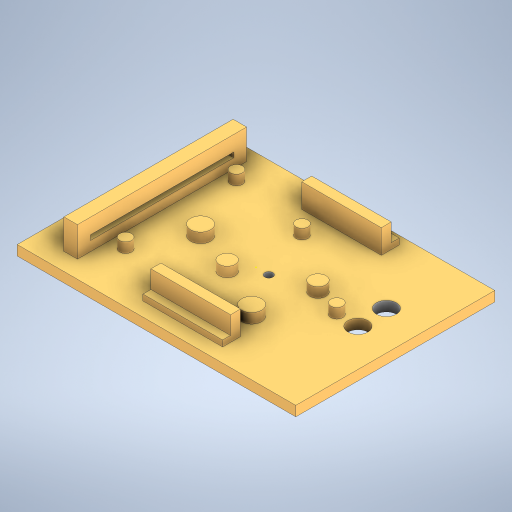
# Autodesk Inventor part: Base
Saved by Autodesk Inventor 2024 (Build 280153000, 153)
## iProperties
Created: 2024-04-22
Part Number: Base
Material: Generic
Document SubType Name: Modeling
Designer: samue
Density: 1 g/cm^3
Appearance: Default
Author: samue
Autodesk Inventor part; units mm, degrees
ref_plane "YZ Plane" through (0, 0, 0) normal (1, 0, 0) x (0, 1, 0)
ref_plane "XZ Plane" through (0, 0, 0) normal (0, 1, 0) x (-1, 0, 0)
ref_plane "XY Plane" through (0, 0, 0) normal (0, 0, 1) x (1, 0, 0)
sketch "Sketch1" plane through (0, 0, 0) normal (0, 1, 0) x (-1, 0, 0)
  line L0 (70, 50) -> (-70, 50)
  line L1 (-70, 50) -> (-70, -50)
  line L2 (-70, -50) -> (70, -50)
  line L3 (70, -50) -> (70, 50)
  line L4 (70, 50) -> (-70, -50) construction
  line L5 (-70, 50) -> (70, -50) construction
  point P0 (0, 0)
  dimension "d0" = 140
  dimension "d1" = 100
  constraints: 12 end point, 2 midpoint, 2 parallel, 1 horizontal, 1 perpendicular
  measures "d0" distance of L2.end L1.end
  measures "d1" distance of L0.end L1.end
extrude "Extrusion1" add sketch "Sketch1" along normal blind 5
sketch "Sketch2" plane through (0, 5, 0) normal (0, 1, 0) x (1, 0, 0)
  circle A0 centre (-42.6045, 32.7902) radius 3
  circle A1 centre (-41.0016, -24.5315) radius 3
  circle A2 centre (-27.8394, 0) radius 5
  circle A3 centre (-2.5867, 25.6769) radius 3
  circle A4 centre (-5.5867, -8.8777) radius 4
  circle A5 centre (19.9874, -22.1936) radius 5
  circle A6 centre (26.1305, 5) radius 4
  circle A7 centre (40.6174, 0) radius 3
  point P0 (0, 0)
  dimension "d4" = 6
  dimension "d5" = 6
  dimension "d6" = 10
  dimension "d7" = 6
  dimension "d8" = 8
  dimension "d9" = 10
  dimension "d12" = 8
  dimension "d13" = 6
  constraints: 8 centre point
  measures "d4" diameter of A0
  measures "d5" diameter of A1
  measures "d6" diameter of A2
  measures "d7" diameter of A3
  measures "d8" diameter of A4
  measures "d9" diameter of A5
  measures "d12" diameter of A6
  measures "d13" diameter of A7
extrude "Extrusion2" add sketch "Sketch2" along normal blind 5
sketch "Sketch3" plane through (0, 5, 0) normal (0, 1, 0) x (1, 0, 0)
  line L0 (-55.5, 43.7813) -> (-48.5, 43.7813)
  line L1 (-48.5, 43.7813) -> (-48.5, -41.2187)
  line L2 (-48.5, -41.2187) -> (-55.5, -41.2187)
  line L3 (-55.5, -41.2187) -> (-55.5, 43.7813)
  line L4 (-70, 50) -> (-70, -50) projected
  point P0 (0, 0)
  dimension "d14" = 7
  dimension "d15" = 85
  dimension "d18" = 21.5
  constraints: 8 end point, 2 parallel, 1 horizontal, 1 perpendicular
  measures "d14" distance of L1.end L2.end
  measures "d15" distance of L0.end L1.end
  measures "d18" distance between parallel lines of L4 L1
extrude "Extrusion3" add sketch "Sketch3" along normal blind 15
sketch "Sketch4" plane through (-48.5, 5, 41.2187) normal (1, 0, 0) x (0, 0, -1)
  line L0 (6.5, 4.85) -> (78.5, 4.85)
  line L1 (78.5, 4.85) -> (78.5, 7.35)
  line L2 (78.5, 7.35) -> (6.5, 7.35)
  line L3 (6.5, 7.35) -> (6.5, 4.85)
  line L4 (85, 0) -> (0, 0) projected
  line L5 (0, 0) -> (0, 15) projected
  point P0 (41.2187, -5)
  dimension "d19" = 2.5
  dimension "d20" = 4.85
  dimension "d23" = 72
  dimension "d24" = 6.5
  constraints: 8 end point, 2 parallel, 1 horizontal, 1 perpendicular
  measures "d19" distance between parallel lines of L2 L0
  measures "d20" distance between parallel lines of L0 L4
  measures "d23" distance of L1.end L2.end
  measures "d24" distance between parallel lines of L5 L3
extrude "Extrusion4" cut sketch "Sketch4" against normal blind 2.5
sketch "Sketch5" plane through (0, 5, 0) normal (0, 1, 0) x (1, 0, 0)
  line L0 (-13.8242, 41.8054) -> (26.1758, 41.8054)
  line L1 (26.1758, 41.8054) -> (26.1758, 36.8054)
  line L2 (26.1758, 36.8054) -> (-13.8242, 36.8054)
  line L3 (-13.8242, 36.8054) -> (-13.8242, 41.8054)
  line L4 (-13.8242, -33.9694) -> (26.1758, -33.9694)
  line L5 (26.1758, -33.9694) -> (26.1758, -38.9694)
  line L6 (26.1758, -38.9694) -> (-13.8242, -38.9694)
  line L7 (-13.8242, -38.9694) -> (-13.8242, -33.9694)
  point P0 (0, 0)
  dimension "d25" = 40
  dimension "d26" = 5
  dimension "d27" = 40
  dimension "d28" = 5
  constraints: 16 end point, 4 parallel, 2 horizontal, 2 perpendicular, 1 point on line
  measures "d25" distance of L1.end L2.end
  measures "d26" distance of L0.end L1.end
  measures "d27" distance of L5.end L6.end
  measures "d28" distance of L4.end L5.end
extrude "Extrusion5" add sketch "Sketch5" along normal blind 12
sketch "Sketch6" plane through (-13.8242, 5, 38.9694) normal (0, 0, 1) x (1, 0, 0)
  line L0 (40, 0) -> (0, 0) projected
  line L1 (0, 0) -> (40, 0)
  line L2 (40, 0) -> (40, 3)
  line L3 (40, 3) -> (0, 3)
  line L4 (0, 3) -> (0, 0)
  point P0 (13.8242, -5)
  dimension "d31" = 40
  dimension "d32" = 3
  constraints: 8 end point, 2 parallel, 1 horizontal, 1 perpendicular
  measures "d31" distance of L3.end L2.end
  measures "d32" distance of L2.end L1.end
extrude "Extrusion6" add sketch "Sketch6" along normal blind 4
sketch "Sketch7" plane through (26.1758, 5, -41.8054) normal (0, 0, -1) x (-1, 0, 0)
  line L0 (40, 0) -> (0, 0) projected
  line L1 (40, 0) -> (40, 12) projected
  line L2 (0, 0) -> (40, 0)
  line L3 (40, 0) -> (40, 3)
  line L4 (40, 3) -> (0, 3)
  line L5 (0, 3) -> (0, 0)
  point P0 (26.1758, -5)
  dimension "d35" = 3
  constraints: 8 end point, 2 parallel, 1 horizontal, 1 perpendicular, 1 point on line
  measures "d35" distance of L3.end L2.end
extrude "Extrusion7" add sketch "Sketch7" along normal blind 4
sketch "Sketch8" plane through (0, 5, 0) normal (0, 1, 0) x (1, 0, 0)
  circle A0 centre (51.2373, 0) radius 5
  point P0 (0, 0)
  dimension "d38" = 10
  constraints: 1 centre point
  measures "d38" diameter of A0
extrude "Extrusion8" cut sketch "Sketch8" against normal blind 8
sketch "Sketch9" plane through (0, 5, 0) normal (0, 1, 0) x (1, 0, 0)
  circle A0 centre (50.6163, 14.9199) radius 5
  point P0 (0, 0)
  dimension "d41" = 10
  constraints: 1 centre point
  measures "d41" diameter of A0
extrude "Extrusion9" cut sketch "Sketch9" against normal blind 10
sketch "Sketch10" plane through (0, 5, 0) normal (0, 1, 0) x (1, 0, 0)
  circle A0 centre (-63.7193, 0) radius 2
  point P0 (0, 0)
  dimension "d44" = 4
  constraints: 1 centre point
  measures "d44" diameter of A0
extrude "Extrusion10" cut sketch "Sketch10" against normal blind 5
sketch "Sketch11" plane through (0, 5, 0) normal (0, 1, 0) x (1, 0, 0)
  circle A0 centre (6.4375, 0) radius 2
  point P0 (0, 0)
  dimension "d47" = 4
  constraints: 1 centre point
  measures "d47" diameter of A0
extrude "Extrusion11" cut sketch "Sketch11" against normal blind 5
sketch "Sketch12" plane through (0, 5, 0) normal (0, 1, 0) x (1, 0, 0)
  point P0 (0, 0)
chamfer "Chamfer1" distance 0.2 angle 45 1 edges at (-55.5, 20, -1.2813)
body "Solid1"
